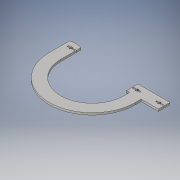
# Autodesk Inventor part: Zoetrope_Hook
Saved by Autodesk Inventor 2016 (Build 200138000, 138)
## iProperties
Created: 2019-03-08
Part Number: Zoetrope_Hook
Material: Generic
Document SubType Name: Modeling
Designer: student
Density: 1 g/cm^3
Appearance: Default
Author: student
Autodesk Inventor part; units mm, degrees
ref_plane "YZ Plane" through (0, 0, 0) normal (1, 0, 0) x (0, 1, 0)
ref_plane "XZ Plane" through (0, 0, 0) normal (0, 1, 0) x (-1, 0, 0)
ref_plane "XY Plane" through (0, 0, 0) normal (0, 0, 1) x (1, 0, 0)
sketch "Sketch1" plane through (0, 0, 0) normal (0, 1, 0) x (-1, 0, 0)
  line L0 (0, 0) -> (114.7109, 0) construction
  line L1 (114.7109, 0) -> (229.0109, 0) construction
  line L2 (63.5, 69.85) -> (63.5, 57.15)
  line L3 (38.1, 69.85) -> (38.1, 57.15)
  arc A0 (203.2, 69.85) -> (63.5, 69.85) centre (133.35, 69.85) ccw
  arc A1 (228.6, 69.85) -> (38.1, 69.85) centre (133.35, 69.85) ccw
  line L4 (229.0109, 0) -> (229.0109, 15.875) construction
  arc A2 (203.2, 25.0136) -> (228.6, 25.0136) centre (215.9, 62.0354) ccw
  line L5 (70.5104, 57.15) -> (63.5, 57.15)
  line L6 (38.1, 57.15) -> (0, 57.15)
  line L7 (70.5104, 43.1165) -> (61.214, 43.1165)
  line L8 (70.5104, 45.7835) -> (61.214, 45.7835)
  line L9 (61.214, 45.7835) -> (61.214, 47.3837)
  line L10 (61.214, 47.3837) -> (58.547, 47.3837)
  line L11 (58.547, 47.3837) -> (58.547, 45.7835)
  line L12 (58.547, 45.7835) -> (52.7304, 45.7835)
  line L13 (52.7304, 45.7835) -> (52.7304, 43.1165)
  line L14 (52.7304, 43.1165) -> (58.547, 43.1165)
  line L15 (58.547, 43.1165) -> (58.547, 41.5163)
  line L16 (58.547, 41.5163) -> (61.214, 41.5163)
  line L17 (61.214, 41.5163) -> (61.214, 43.1165)
  line L18 (70.5104, 45.7835) -> (70.5104, 57.15)
  line L19 (70.5104, 43.1165) -> (70.5104, 31.75)
  line L20 (70.5104, 31.75) -> (0, 31.75)
  line L21 (0, 43.1165) -> (9.2964, 43.1165)
  line L22 (0, 45.7835) -> (9.2964, 45.7835)
  line L23 (9.2964, 45.7835) -> (9.2964, 47.3837)
  line L24 (9.2964, 47.3837) -> (11.9634, 47.3837)
  line L25 (11.9634, 47.3837) -> (11.9634, 45.7835)
  line L26 (11.9634, 45.7835) -> (17.78, 45.7835)
  line L27 (17.78, 45.7835) -> (17.78, 43.1165)
  line L28 (17.78, 43.1165) -> (11.9634, 43.1165)
  line L29 (11.9634, 43.1165) -> (11.9634, 41.5163)
  line L30 (11.9634, 41.5163) -> (9.2964, 41.5163)
  line L31 (9.2964, 41.5163) -> (9.2964, 43.1165)
  line L32 (0, 57.15) -> (0, 45.7835)
  line L33 (0, 43.1165) -> (0, 31.75)
  line L34 (203.2, 38.0368) -> (212.4964, 38.0368)
  line L35 (212.4964, 38.0368) -> (212.4964, 39.637)
  line L36 (212.4964, 39.637) -> (215.1634, 39.637)
  line L37 (215.1634, 39.637) -> (215.1634, 38.0368)
  line L38 (215.1634, 38.0368) -> (220.98, 38.0368)
  line L39 (220.98, 38.0368) -> (220.98, 35.3698)
  line L40 (220.98, 35.3698) -> (215.1634, 35.3698)
  line L41 (215.1634, 35.3698) -> (215.1634, 33.7696)
  line L42 (215.1634, 33.7696) -> (212.4964, 33.7696)
  line L43 (212.4964, 33.7696) -> (212.4964, 35.3698)
  line L44 (212.4964, 35.3698) -> (203.2, 35.3698)
  line L45 (228.6, 69.85) -> (228.6, 25.0136)
  line L46 (203.2, 25.0136) -> (203.2, 35.3698)
  line L47 (203.2, 69.85) -> (203.2, 38.0368)
  dimension "d12" = 12.7
  dimension "d16" = 25.4
  dimension "d19" = 190.5
  dimension "d20" = 15.875
  dimension "d38" = 95.25
  dimension "d48" = 70.5104
  dimension "d53" = 9.2964
  dimension "d54" = 1.6002
  dimension "d55" = 2.667
  dimension "d56" = 5.8166
  dimension "d57" = 1.6002
  dimension "d58" = 9.2964
  dimension "d59" = 2.667
  dimension "d60" = 5.8166
  dimension "d61" = 1.6002
  dimension "d62" = 37.868
  dimension "d63" = 12.7
  dimension "d64" = 22.3984
  dimension "d66" = 2.667
  dimension "d67" = 11.3665
  dimension "d68" = 11.3665
  dimension "d69" = 11.3665
  dimension "d70" = 11.3665
  dimension "d71" = 38.1
  constraints: 96 end point, 12 perpendicular, 10 horizontal, 10 vertical, 7 point on line, 6 point on circle, 3 centre point, 2 tangent, 1 parallel
  measures "d12" distance of L2.start L2.end
  measures "d16" distance between parallel lines of L3 L2
  measures "d19" distance of L3.start L45.start
  measures "d20" distance of L1.end L4.end
  measures "d38" radius of A1
  measures "d48" distance of L20.end L19.end
  measures "d53" distance of L7.start L7.end
  measures "d54" distance of L8.end L9.end
  measures "d55" distance of L9.end L10.end
  measures "d56" distance of L11.end L12.end
  measures "d57" distance of L14.end L15.end
  measures "d58" distance of L34.start L34.end
  measures "d59" distance of L35.end L36.end
  measures "d60" distance of L37.end L38.end
  measures "d61" distance of L40.end L41.end
  measures "d63" distance from line of L45 A2.centre
  measures "d64" distance from line of A2.centre L36
  measures "d66" distance of L38.end L39.end
  measures "d67" distance of L8.start L5.start
  measures "d68" distance of L7.start L19.end
  measures "d69" distance of L6.end L22.start
  measures "d70" distance of L21.start L20.end
  measures "d71" distance of L3.end L6.end
extrude "Extrusion2" add sketch "Sketch1" along normal blind 4.572
body "Solid2"
